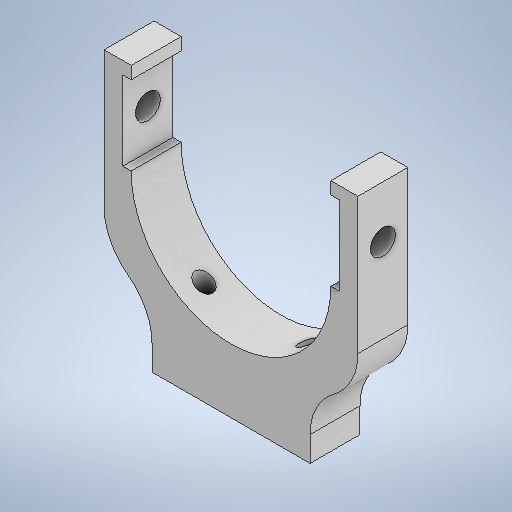
# Autodesk Inventor part: 102
Saved by Autodesk Inventor 2025.1 (Build 291241000, 241)
## iProperties
Created: 2024-06-10
Part Number: 102
Material: Generisch
Document SubType Name: Modeling
Designer: ffogue
Density: 1 g/cm^3
Appearance: Vorgabe
Author: ffogue
Autodesk Inventor part; units mm, degrees
ref_plane "YZ Plane" through (0, 0, 0) normal (1, 0, 0) x (0, 1, 0)
ref_plane "XZ Plane" through (0, 0, 0) normal (0, 1, 0) x (-1, 0, 0)
ref_plane "XY Plane" through (0, 0, 0) normal (0, 0, 1) x (1, 0, 0)
sketch "Skizze1" plane through (0, 0, 0) normal (0, 1, 0) x (-1, 0, 0)
  line L0 (54.5, 0) -> (61, 0)
  line L1 (61, 0) -> (61, -32.7433)
  arc A0 (55.25, -44.0542) -> (61, -32.7433) centre (47, -32.7433) ccw
  arc A1 (55.25, -44.0542) -> (49.5, -55.3652) centre (63.5, -55.3652) ccw
  line L2 (54.5, 0) -> (54.5, -2.9933)
  line L3 (54.5, -2.9933) -> (56.5, -2.9933)
  line L4 (56.5, -2.9933) -> (56.5, -21.9933)
  line L5 (56.5, -21.9933) -> (54.5, -21.9933)
  arc A2 (6.5, -21.9933) -> (54.5, -21.9933) centre (30.5, -21.9933) ccw
  arc A3 (11.5, -55.3652) -> (5.75, -44.0542) centre (-2.5, -55.3652) ccw
  arc A4 (0, -32.7433) -> (5.75, -44.0542) centre (14, -32.7433) ccw
  line L6 (0, -32.7433) -> (0, 0)
  line L7 (0, 0) -> (6.5, 0)
  line L8 (6.5, 0) -> (6.5, -2.9933)
  line L9 (6.5, -2.9933) -> (4.5, -2.9933)
  line L10 (4.5, -2.9933) -> (4.5, -21.9933)
  line L11 (4.5, -21.9933) -> (6.5, -21.9933)
  line L12 (11.5, -55.3652) -> (11.5, -61.3652)
  line L13 (11.5, -61.3652) -> (49.5, -61.3652)
  line L14 (49.5, -61.3652) -> (49.5, -55.3652)
  line L15 (49.5, -55.3652) -> (49.5, -61.3652)
  line L16 (30.5, -51.8632) -> (30.5, -31.0026) construction
  point P0 (54.5, -1.4967)
  point P1 (6.5, -1.4967)
  point P2 (30.5, -21.9933)
  point P3 (30.5, -61.3652)
  point P4 (56.5, -12.4933)
  dimension "d2" = 2
  dimension "d3" = 19
  dimension "d4" = 14
  dimension "d5" = 14
  dimension "d6" = 38
  dimension "d10" = 19
  dimension "d12" = 2
  dimension "d13" = 24
  dimension "d14" = 24
  dimension "d18" = 4.5
  dimension "d19" = 4.5
  dimension "d20" = 24
  dimension "d54" = 19
  dimension "d55" = 6
  dimension "d56" = 14
  dimension "d57" = 14
  dimension "d58" = 42.8719
  dimension "d59" = 10.75
  constraints: 34 end point, 11 perpendicular, 10 point on circle, 6 tangent, 5 centre point, 4 midpoint, 4 vertical, 3 horizontal alignment, 2 coincident, 2 point on line, 2 vertical alignment, 1 collinear, 1 horizontal
  measures "d2" distance from line of point (54.5, -1.497) L4
  measures "d3" distance of L3.end L4.end
  measures "d4" radius of A0
  measures "d5" radius of A1
  measures "d6" distance of L14.end L12.start
  measures "d10" distance of L9.end L10.end
  measures "d12" distance from line of L10 point (6.5, -1.497)
  measures "d13" distance from line of A2.centre L2
  measures "d14" distance from line of A2.centre L8
  measures "d18" distance between parallel lines of L6 L10
  measures "d19" distance between parallel lines of L4 L1
  measures "d20" radius of A2
  measures "d54" distance from line of L14 point (30.5, -61.365)
  measures "d55" distance from line of L13 A1.centre
  measures "d56" radius of A3
  measures "d57" radius of A4
  measures "d58" vertical distance of A1.centre point (56.5, -12.493)
  measures "d59" vertical distance of A0.centre A2.centre
extrude "Extrusion1" add sketch "Skizze1" along normal blind 12
sketch "Skizze2" plane through (-11.5, 0, -61.3652) normal (0, 0, -1) x (-1, 0, 0)
  line L0 (0, 0) -> (0, 12) projected
  line L1 (0, 0) -> (38, 0) projected
  point P0 (-11.5, 0)
  point P1 (6.5, 6)
  point P2 (31.5, 6)
  point P3 (0, 6)
  point P4 (19, 0)
  dimension "d35" = 25
  dimension "d36" = 12.5
  constraints: 2 horizontal alignment, 2 midpoint
  measures "d35" distance of point (31.5, 6) point (6.5, 6)
  measures "d36" horizontal distance of point (19, 0) point (6.5, 6)
hole "Bohrung1" at (-18, 6, -61.3652) at (-43, 6, -61.3652) direction (0, 0, 1) diameter 4.134 end through all thread size "M5x0.8" class "6H" standard "ISO Metric profile"
sketch "Skizze3" plane through (0, 0, 0) normal (1, 0, 0) x (0, 0, -1)
  line L0 (0, 0) -> (0, 12) projected
  point P0 (12.5, 6)
  point P1 (0, 6)
  dimension "d44" = 12.5
  constraints: 1 horizontal alignment, 1 midpoint
  measures "d44" distance from line of L0 point (12.5, 6)
hole "Bohrung2" at (0, 6, -12.5) direction (1, 0, 0) diameter 6 depth 4.5
sketch "Skizze4" plane through (-61, 0, -32.7433) normal (-1, 0, 0) x (0, 0, 1)
  line L0 (32.7433, 0) -> (32.7433, 12) projected
  point P0 (20.2433, 6)
  point P1 (32.7433, 6)
  dimension "d53" = 12.5
  constraints: 1 horizontal alignment, 1 midpoint
  measures "d53" distance from line of point (20.243, 6) L0
hole "Bohrung3" at (-61, 6, -12.5) direction (1, 0, 0) diameter 6 end through all
equation "\"d10\" = d3"
equation "\"d19\" = d18"
